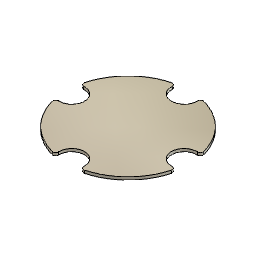
temperature diode contact CAM v5 (Autodesk Fusion 360 archive; units mm, degrees)
design "silver contact part"
Autodesk Fusion 360 part; units mm, degrees
sketch "Sketch1" plane through (0, 0, 0) normal (0, 1, 0) x (1, 0, 0)
  circle A0 centre (0, 0) radius 10 construction
  circle A1 centre (10, 0) radius 2.25
  circle A2 centre (0, 10) radius 2.25
  circle A3 centre (-10, 0) radius 2.25
  circle A4 centre (0, -10) radius 2.25
  circle A5 centre (0, 0) radius 11
  dimension "d1" = 20
  dimension "d2" = 4.5
  dimension "d4" = 360
  dimension "d5" = 22
  constraint coincident A0.centre A5.centre
  constraint coincident A0 A1.centre
  constraint horizontal A0.centre A1.centre
  constraint concentric A0 A5
  measures "d1" diameter of A0
  measures "d2" diameter of A1
  measures "d5" diameter of A5
extrude "Extrude1" add sketch "Sketch1" along normal blind 0.5 contours A1 A2 A3 A4 A5
fillet "Fillet1" radius 0.5 8 edges at (-2.1042, 0.25, 10.7969) (2.1042, 0.25, 10.7969) (-10.7969, 0.25, 2.1042) (-10.7969, 0.25, -2.1042) (-2.1042, 0.25, -10.7969) (2.1042, 0.25, -10.7969) (10.7969, 0.25, -2.1042) (10.7969, 0.25, 2.1042)

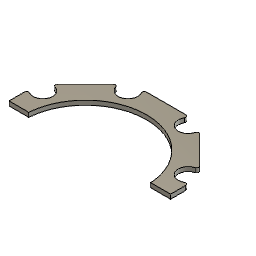
design "stage 1 shield pressure clamp"
Autodesk Fusion 360 part; units mm, degrees
sketch "Sketch1" plane through (0, 0, 0) normal (0, 1, 0) x (1, 0, 0)
  circle A0 centre (0, 0) radius 18 construction
  circle A1 centre (0, 0) radius 14
  circle A2 centre (-16.6298, 6.8883) radius 2.25
  circle A3 centre (-16.6298, -6.8883) radius 2.25
  circle A4 centre (-6.8883, -16.6298) radius 2.25
  circle A5 centre (6.8883, -16.6298) radius 2.25
  circle A6 centre (16.6298, -6.8883) radius 2.25
  circle A7 centre (16.6298, 6.8883) radius 2.25
  circle A8 centre (6.8883, 16.6298) radius 2.25
  circle A9 centre (-6.8883, 16.6298) radius 2.25
  line L0 (-18.5, 7.663) -> (-18.5, -7.663)
  line L1 (-18.5, -7.663) -> (-7.663, -18.5)
  line L2 (-7.663, -18.5) -> (7.663, -18.5)
  line L3 (7.663, -18.5) -> (18.5, -7.663)
  line L4 (18.5, -7.663) -> (18.5, 7.663)
  line L5 (18.5, 7.663) -> (7.663, 18.5)
  line L6 (7.663, 18.5) -> (-7.663, 18.5)
  line L7 (-7.663, 18.5) -> (-18.5, 7.663)
  line L8 (-18.5, 1) -> (18.5, 1)
  point P0 (-16.6298, 6.8883)
  dimension "d1" = 36
  dimension "d2" = 28
  dimension "d3" = 4.5
  dimension "d5" = 360
  dimension "d6" = 18.5
  dimension "d7" = 1
  constraint coincident A0.centre A1.centre
  constraint concentric A0 A1
  constraint coincident A0 P0
  constraint coincident P0 A2.centre
  constraint horizontal A8.centre A9.centre
  constraint horizontal L6
  constraint coincident L0 L8.start
  constraint coincident L4 L8.end
  constraint perpendicular L4 L8
  measures "d1" diameter of A0
  measures "d2" diameter of A1
  measures "d3" diameter of A2
  measures "d6" distance of A0.centre L7
  measures "d7" distance of A0.centre L8
extrude "Extrude1" add sketch "Sketch1" along normal blind 1 contours A1 A2 A7 A8 A9 L0 L4 L5 L6 L7 L8
fillet "Fillet1" radius 0.5 8 edges at (18.5, 0.5, -5.6373) (17.0677, 0.5, -9.0953) (9.0953, 0.5, -17.0677) (5.6373, 0.5, -18.5) (-5.6373, 0.5, -18.5) (-9.0953, 0.5, -17.0677) (-17.0677, 0.5, -9.0953) (-18.5, 0.5, -5.6373)

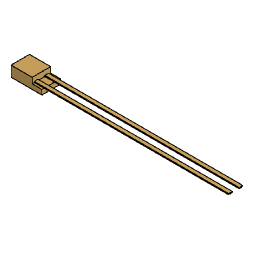
design "Lakeshore DT 670 SD Omega CY 670 SD"
Autodesk Fusion 360 part; units mm, degrees
sketch "Sketch1" plane through (0, 0, 0) normal (0, 0, 1) x (1, 0, 0)
  line L0 (0, 0) -> (3.175, 0)
  line L1 (3.175, 0) -> (3.175, 0.5)
  line L2 (3.175, 0.5) -> (2.175, 0.5)
  line L3 (2.175, 0.5) -> (2.175, 1.08)
  line L4 (2.175, 1.08) -> (0, 1.08)
  line L5 (0, 1.08) -> (0, 0)
  dimension "d1" = 1.08
  dimension "d2" = 3.175
  dimension "d3" = 1
  dimension "d4" = 0.5
  constraint coincident L0.start L5.end
  constraint horizontal L0
  constraint perpendicular L0 L1
  constraint perpendicular L1 L2
  constraint perpendicular L0 L3
  constraint perpendicular L3 L4
  constraint perpendicular L0 L5
  measures "d1" distance of L4.end L0.start
  measures "d2" distance of L0.start L0.end
  measures "d3" distance of L1.end L2.end
  measures "d4" distance of L0.end L1.end
extrude "Extrude1" add sketch "Sketch1" along normal blind 1.905
sketch "Sketch2" plane through (0, 0.5, 0) normal (0, 1, 0) x (-1, 0, 0)
  line L0 (-3.175, 0) -> (-2.175, 0)
  line L1 (-2.175, 0) -> (-2.175, 1.905)
  line L2 (-2.175, 1.905) -> (-3.175, 1.905)
  line L3 (-3.175, 1.905) -> (-3.175, 0)
  line L4 (-2.175, 0.2225) -> (-22.175, 0.2225)
  line L5 (-22.175, 0.2225) -> (-22.175, 0.6035)
  line L6 (-22.175, 0.6035) -> (-2.175, 0.6035)
  line L7 (-2.175, 0.6035) -> (-2.175, 0.2225)
  line L8 (-3.175, 0.9525) -> (0, 0.9525) construction
  line L9 (-2.175, 1.6825) -> (-22.175, 1.6825)
  line L10 (-22.175, 1.3015) -> (-2.175, 1.3015)
  line L11 (-22.175, 1.6825) -> (-22.175, 1.3015)
  line L12 (-2.175, 1.3015) -> (-2.175, 1.6825)
  dimension "d7" = 0.381
  dimension "d8" = 19
  dimension "d9" = 0.698
  constraint horizontal L4
  constraint vertical L5
  constraint horizontal L6
  constraint vertical L7
  constraint collinear L1 L7
  constraint midpoint L3 L8.start
  constraint perpendicular L3 L8
  constraint symmetric L4.start L8 L9.start
  constraint symmetric L4.end L8 L9.end
  constraint symmetric L5.end L8 L10.start
  constraint symmetric L6.end L8 L10.end
  measures "d7" distance of L4.end L5.end
  measures "d8" distance of L3 L5
  measures "d9" distance of L6 L10
extrude "Extrude2" add sketch "Sketch2" along normal blind 0.102 contours L3 L4 L5 L6 | L1 L3 L4 L6 L7 | L3 L9 L10 L11 | L1 L3 L9 L10 L12

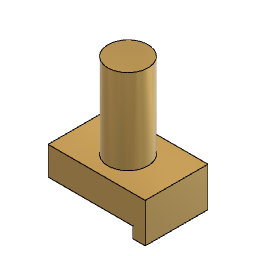
design "Lakeshore CO clamp"
Autodesk Fusion 360 part; units mm, degrees
sketch "Sketch1" plane through (0, 0, 0) normal (0, 0, 1) x (1, 0, 0)
  line L0 (0, 0) -> (0, 3.2)
  line L1 (0, 3.2) -> (-7.9, 3.2)
  line L2 (-7.9, 3.2) -> (-7.9, 0.9)
  line L3 (-7.9, 0.9) -> (-1, 0.9)
  line L4 (-1, 0.9) -> (-1, 0)
  line L5 (-1, 0) -> (0, 0)
  dimension "d1" = 3.2
  dimension "d2" = 7.9
  dimension "d3" = 0.9
  dimension "d4" = 1
  constraint coincident L0.start L5.end
  constraint vertical L0
  constraint perpendicular L0 L1
  constraint perpendicular L1 L2
  constraint perpendicular L2 L3
  constraint perpendicular L1 L4
  constraint perpendicular L0 L5
  measures "d1" distance of L0.start L0.end
  measures "d2" distance of L0.end L1.end
  measures "d3" distance of L3.end L4.end
  measures "d4" distance of L4.end L0.start
extrude "Extrude1" add sketch "Sketch1" along normal blind 5.1
hole "Hole1" at (-3.95, 3.2, 2.55) direction (0, -1, 0) diameter 3.264 depth 5 tip angle 118
sketch "Sketch2" plane through (0, 0, 0) normal (0, 1, 0) x (1, 0, 0)
  circle A0 centre (-3.95, -2.55) radius 2
  circle A1 centre (-3.95, -2.55) radius 1.632
  dimension "d10" = 4
  constraint concentric A0 A1
  measures "d10" diameter of A0
extrude "Extrude2" add sketch "Sketch2" along normal up to surface (10.1 mm away) contours A1
